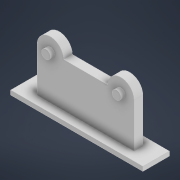
# Autodesk Inventor part: Base
Saved by Autodesk Inventor 2021.2 (Build 252289000, 289)
## iProperties
Created: 2021-05-30
Part Number: Base
Material: Типовые
Document SubType Name: Modeling
Designer: Admin
Density: 1 g/cm^3
Appearance: По умолчанию
Author: Admin
Autodesk Inventor part; units mm, degrees
ref_plane "YZ Plane" through (0, 0, 0) normal (1, 0, 0) x (0, 1, 0)
ref_plane "XZ Plane" through (0, 0, 0) normal (0, 1, 0) x (-1, 0, 0)
ref_plane "XY Plane" through (0, 0, 0) normal (0, 0, 1) x (1, 0, 0)
sketch "Эскиз1" plane through (0, 0, 0) normal (0, 1, 0) x (-1, 0, 0)
  line L0 (0, 0) -> (-150, 0)
  line L1 (-150, 0) -> (-150, -30)
  line L2 (-150, -30) -> (0, -30)
  line L3 (0, -30) -> (0, 0)
  dimension "d0" = 150
  dimension "d1" = 30
  constraints: 8 end point, 2 parallel, 1 horizontal, 1 perpendicular
  measures "d0" distance of L2.end L1.end
  measures "d1" distance of L1.end L0.end
extrude "Выдавливание1" add sketch "Эскиз1" along normal blind 5
sketch "Эскиз3" plane through (0, 5, 0) normal (0, 1, 0) x (1, 0, 0)
  line L0 (20, 20) -> (130, 20)
  line L1 (130, 20) -> (130, 10)
  line L2 (130, 10) -> (20, 10)
  line L3 (20, 10) -> (20, 20)
  line L4 (150, 30) -> (0, 30) projected
  line L5 (0, 0) -> (150, 0) projected
  line L6 (0, 30) -> (0, 0) projected
  line L7 (150, 0) -> (150, 30) projected
  dimension "d8" = 10
  dimension "d9" = 10
  dimension "d10" = 20
  dimension "d11" = 20
  constraints: 8 end point, 2 parallel, 1 horizontal, 1 perpendicular
  measures "d8" distance between parallel lines of L4 L0
  measures "d9" distance between parallel lines of L5 L2
  measures "d10" distance between parallel lines of L6 L3
  measures "d11" distance between parallel lines of L7 L1
extrude "Выдавливание3" add sketch "Эскиз3" along normal blind 50 contours L0 L1 L2 L3
sketch "Эскиз4" plane through (20, 5, -10) normal (0, 0, 1) x (1, 0, 0)
  arc A0 (30, 50) -> (0, 50) centre (15, 50) ccw
  line L0 (0, 50) -> (110, 50) projected
  line L1 (0, 0) -> (0, 50) projected
  line L2 (55, 50) -> (55, 234.7508)
  arc A1 (110, 50) -> (80, 50) centre (95, 50) ccw
  point P0 (-20, -5)
  dimension "d14" = 30
  constraints: 4 point on circle, 3 end point, 2 centre point, 2 point on line, 2 symmetric about line, 1 midpoint, 1 tangent, 1 vertical, 1 other
  measures "d14" diameter of A0
extrude "Выдавливание4" add sketch "Эскиз4" against normal up to surface (10 mm away)
sketch "Эскиз5" plane through (20, 5, -10) normal (0, 0, 1) x (1, 0, 0)
  arc A0 (30, 50) -> (0, 50) centre (15, 50) ccw projected
  arc A1 (110, 50) -> (80, 50) centre (95, 50) ccw projected
  circle A2 centre (15, 50) radius 5
  circle A3 centre (95, 50) radius 5
  point P0 (-20, -5)
  point P1 (55, 199.7494)
  dimension "d24" = 10
  dimension "d25" = 10
  constraints: 4 coincident, 2 centre point
  measures "d24" diameter of A2
  measures "d25" diameter of A3
extrude "Выдавливание5" add sketch "Эскиз5" along normal blind 5
